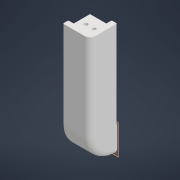
# Autodesk Inventor part: frame-foot
Saved by Autodesk Inventor 2021 (Build 250183000, 183)
## iProperties
Created: 2020-05-09
Part Number: frame-foot
Material: Generic
Document SubType Name: Modeling
Designer: Jonathan
Density: 1 g/cm^3
Appearance: Default
Author: Jonathan
Autodesk Inventor part; units mm, degrees
ref_plane "YZ Plane" through (0, 0, 0) normal (1, 0, 0) x (0, 1, 0)
ref_plane "XZ Plane" through (0, 0, 0) normal (0, 1, 0) x (-1, 0, 0)
ref_plane "XY Plane" through (0, 0, 0) normal (0, 0, 1) x (1, 0, 0)
ref_plane "Work Plane1" through (0, 0, 0) normal (0, 0, 1) x (1, 0, 0)
sketch "Sketch1" plane through (0, 0, 0) normal (0, 0, 1) x (1, 0, 0)
  arc A0 (12.5, 11.5) -> (11.5, 12.5) centre (11.5, 11.5) ccw projected
  line L0 (8.5, 12.5) -> (11.5, 12.5) projected
  arc A1 (8.5, 12.5) -> (7.5, 11.5) centre (8.5, 11.5) ccw projected
  line L1 (7.5, 1.5) -> (7.5, 11.5) projected
  arc A2 (-12.5, -11.5) -> (-11.5, -12.5) centre (-11.5, -11.5) ccw projected
  line L2 (7.5, -12.5) -> (-11.5, -12.5) projected
  arc A3 (7.5, -12.5) -> (12.5, -7.5) centre (7.5, -7.5) ccw projected
  line L3 (12.5, 11.5) -> (12.5, -7.5) projected
  arc A4 (-11.5, 1.5) -> (-12.5, 0.5) centre (-11.5, 0.5) ccw projected
  line L4 (-12.5, 0.5) -> (-12.5, -11.5) projected
  line L5 (7.5, 1.5) -> (-11.5, 1.5) projected
  circle A5 centre (-2.5, -3) radius 1.65 projected
  arc A6 (12.5, 11.5) -> (11.5, 12.5) centre (11.5, 11.5) ccw projected
  line L6 (12.5, -7.5) -> (12.5, 11.5) projected
  arc A7 (7.5, -12.5) -> (12.5, -7.5) centre (7.5, -7.5) ccw projected
  line L7 (1.0011, -12.5) -> (7.5, -12.5) projected
  line L8 (-6.0011, -12.5) -> (1.0011, -12.5) projected
  line L9 (-11.5, -12.5) -> (-6.0011, -12.5) projected
  arc A8 (-12.5, -11.5) -> (-11.5, -12.5) centre (-11.5, -11.5) ccw projected
  line L10 (-12.5, -8.5) -> (-12.5, -11.5) projected
  arc A9 (-11.5, -7.5) -> (-12.5, -8.5) centre (-11.5, -8.5) ccw projected
  line L11 (2.5, -7.5) -> (-11.5, -7.5) projected
  arc A10 (2.5, -7.5) -> (7.5, -2.5) centre (2.5, -2.5) ccw projected
  line L12 (7.5, 11.5) -> (7.5, -2.5) projected
  arc A11 (8.5, 12.5) -> (7.5, 11.5) centre (8.5, 11.5) ccw projected
  line L13 (8.5, 12.5) -> (11.5, 12.5) projected
revolve "Revolution1" add sketch "Sketch1" angle 90 about axis through (8.5, 12.5, 0) along (-1, 0, 0) contours L3 A3 L2 A2 L4 A9 L11 A10 L12 L1 A1 L0 A0
sketch "Sketch2" plane through (8.5, 12.5, 0) normal (0, 1, 0) x (1, 0, 0)
  line L0 (4, -20) -> (4, -1) projected
  arc A0 (4, -1) -> (3, 0) centre (3, -1) ccw projected
  line L1 (3, 0) -> (0, 0) projected
  arc A1 (0, 0) -> (-1, -1) centre (0, -1) ccw projected
  line L2 (-1, -1) -> (-1, -15) projected
  arc A2 (-21, -24) -> (-20, -25) centre (-20, -24) ccw projected
  line L3 (-20, -25) -> (-1, -25) projected
  arc A3 (-1, -25) -> (4, -20) centre (-1, -20) ccw projected
  line L4 (-21, -21) -> (-21, -24) projected
  line L5 (-6, -20) -> (-20, -20) projected
  arc A4 (-20, -20) -> (-21, -21) centre (-20, -21) ccw projected
  arc A5 (-6, -20) -> (-1, -15) centre (-6, -15) ccw projected
  point P0 (-8.5, 0)
extrude "Extrusion1" add sketch "Sketch2" along normal up to surface (79.8139 mm away)
sketch "Sketch5" plane through (7.5, -12.5, 0) normal (0, 0, -1) x (-1, 0, 0)
  line L0 (20, 99.8139) -> (-1, 99.8139)
  line L1 (-1, 99.8139) -> (-1, 94.8139)
  line L2 (-1, 94.8139) -> (20, 94.8139)
  line L3 (20, 94.8139) -> (20, 99.8139)
  line L4 (20, 25) -> (20, 104.8139) projected
  line L5 (19, 104.8139) -> (5, 104.8139) projected
  point P0 (7.5, 12.5)
  point P1 (-1, 104.8139)
  dimension "d10" = 5
  dimension "d11" = 5
  constraints: 8 end point, 2 parallel, 2 point on line, 1 horizontal, 1 perpendicular
  measures "d10" distance between parallel lines of L5 L0
  measures "d11" distance between parallel lines of L0 L2
extrude "Extrusion4" add sketch "Sketch5" against normal up to next
sketch "Sketch6" plane through (-12.5, 82.3139, 0) normal (0, -1, 0) x (1, 0, 0)
  circle A0 centre (13.75, 10) radius 1.65
  circle A1 centre (6.25, 10) radius 1.65
  line L0 (13.75, 10) -> (6.25, 10) construction
  line L1 (20, 15) -> (20, 1) projected
  line L2 (20, 2.0913) -> (0, 2.0913) construction
  line L3 (21, 0) -> (0, 0) projected
  line L4 (10, 0) -> (10, 20) construction
  line L5 (1, 20) -> (15, 20) projected
  line L6 (0, 0) -> (0, 21) projected
  point P0 (12.5, 0)
  point P1 (10, 2.0913)
  point P2 (10, 10)
  point P3 (20, 11)
  point P4 (0, 12)
  dimension "d14" = 7.5
  dimension "d15" = 3.3
  constraints: 6 end point, 5 point on line, 3 midpoint, 2 centre point, 2 horizontal, 1 equal radius, 1 horizontal alignment, 1 vertical
  measures "d14" distance of L0.end L0.start
  measures "d15" diameter of A0
extrude "Extrusion5" cut sketch "Sketch6" against normal through all
sketch "Sketch8" plane through (7.5, -12.5, 0) normal (0, 0, -1) x (-1, 0, 0)
  arc A0 (20, 4) -> (19, 5) centre (19, 4) ccw projected
  line L0 (-1, 25) -> (-1, 94.8139) projected
  line L1 (20, 4) -> (-1, 4)
  line L2 (-1, 4) -> (-1, 14)
  line L3 (-1, 14) -> (20, 14)
  line L4 (20, 14) -> (20, 4)
  point P0 (7.5, 12.5)
  dimension "d18" = 10
  constraints: 8 end point, 2 parallel, 1 horizontal, 1 perpendicular, 1 point on line
  measures "d18" distance of L3.end L1.start
extrude "Extrusion6" add sketch "Sketch8" against normal up to next
sketch "Sketch9" plane through (7.5, -12.5, 0) normal (0, 0, -1) x (-1, 0, 0)
  circle A0 centre (10, 9.5) radius 1.65
  arc A1 (-4, 25) -> (-5, 24) centre (-4, 24) ccw projected
  line L0 (-1, 25) -> (-4, 25) projected
  arc A2 (0, 24) -> (-1, 25) centre (-1, 24) ccw projected
  line L1 (0, 14) -> (0, 24) projected
  arc A3 (19, 0) -> (20, 1) centre (19, 1) ccw projected
  line L2 (0, 0) -> (19, 0) projected
  arc A4 (-5, 5) -> (0, 0) centre (0, 5) ccw projected
  line L3 (-5, 24) -> (-5, 5) projected
  line L4 (20, 1) -> (20, 14) projected
  line L5 (20, 9.5) -> (0, 9.5) construction
  line L6 (10, 5) -> (10, 14) construction
  line L7 (20, 14) -> (0, 14) projected
  arc A5 (20, 13) -> (19, 14) centre (19, 13) ccw projected
  line L8 (20, 13) -> (20, 1) projected
  line L9 (0, 14) -> (19, 14) projected
  circle A6 centre (10, 9.5) radius 1.65 projected
  point P0 (7.5, 12.5)
  point P1 (20, 4)
  point P2 (10, 9.5)
  dimension "d21" = 3.3
  constraints: 4 end point, 3 midpoint, 2 point on line, 1 centre point, 1 coincident, 1 perpendicular, 1 vertical
  measures "d21" diameter of A0
extrude "Extrusion7" cut sketch "Sketch9" against normal blind 10 contours A0
sketch "Sketch11" plane through (-2.5, -3, 10) normal (0, 0, -1) x (-1, 0, 0)
  line L0 (0, -3.3486) -> (-2.9, -1.6743)
  line L1 (-2.9, -1.6743) -> (-2.9, 1.6743)
  line L2 (-2.9, 1.6743) -> (0, 3.3486)
  line L3 (0, 3.3486) -> (2.9, 1.6743)
  line L4 (2.9, 1.6743) -> (2.9, -1.6743)
  line L5 (2.9, -1.6743) -> (0, -3.3486)
  line L6 (0, 6.2514) -> (0, -6.2514) construction
  circle A0 centre (0, 0) radius 1.65 construction
  circle A1 centre (0, 0) radius 1.65
  point P0 (-2.5, 3)
  dimension "d27" = 9.6
  dimension "d28" = 5.8
  constraints: 14 end point, 3 coincident, 1 centre point, 1 midpoint, 1 point on line, 1 vertical, 13 other
  measures "d27" distance of L6.start L0.start
  measures "d28" distance between parallel lines of L0 L3
extrude "Extrusion8" cut sketch "Sketch11" along normal blind 2.7
sketch "Sketch12" plane through (-12.5, 1.5, 0) normal (0, 1, 0) x (1, 0, 0)
  line L0 (7.1, -10) -> (10, -10) projected
  line L1 (10, -10) -> (12.9, -10) projected
  line L2 (12.9, -10) -> (10, -10) projected
  line L3 (10, -10) -> (7.1, -10) projected
  line L4 (7.1, -10) -> (7.1, -7.3)
  line L5 (7.1, -10) -> (7.1, -7.3) projected
  line L6 (7.1, -7.3) -> (12.9, -7.3)
  line L7 (12.9, -10) -> (12.9, -7.3) projected
  line L8 (12.9, -7.3) -> (12.9, -10)
  point P0 (12.5, 0)
  dimension "d31" = 2.7
  constraints: 6 end point, 2 collinear, 1 perpendicular
  measures "d31" distance of L0.start L4.end
extrude "Extrusion9" cut sketch "Sketch12" against normal up to next
sketch "Sketch13" plane through (7.5, -12.5, 10) normal (0, 0, -1) x (-1, 0, 0)
  circle A0 centre (10, 9.5) radius 1.65 projected
  circle A1 centre (10, 9.5) radius 1.65
  point P0 (7.5, 12.5)
  constraints: 1 centre point, 1 coincident
extrude "Extrusion10" cut sketch "Sketch13" against normal blind 5
body "Solid1"
